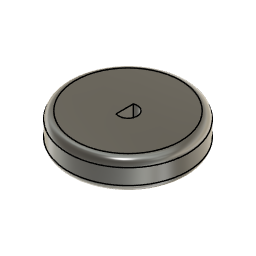
wheel v2 v1 (Autodesk Fusion 360 design; units mm, degrees)
Autodesk Fusion 360 part; units mm, degrees
note: some values were not read from the file. Set by a fixed rule: which sketch regions a step uses.
sketch "Sketch1" plane through (0, 0, 0) normal (0, 0, 1) x (1, 0, 0)
  circle A0 centre (0, 0) radius 10
  dimension "d1" = 20
  constraint coincident A0.centre origin
  measures "d1" diameter of A0
extrude "Extrude1" add sketch "Sketch1" along normal blind 5
fillet "Fillet1" radius 1.2 2 edges at (-9.3233, -3.6162, 5) (-9.3233, -3.6162, 0)
sketch "Sketch2" plane through (0, 0, 5) normal (0, 0, 1) x (-1, 0, 0)
  circle A0 centre (0, 0) radius 8.8
  circle A1 centre (0, 0) radius 1.55
  line L0 (0.55, 1.4491) -> (2.3002, 1.4491)
  line L1 (2.3002, 1.4491) -> (2.3002, -1.4465)
  line L2 (2.3002, -1.4465) -> (0.55, -1.4465)
  line L3 (0.55, -1.4465) -> (0.55, 1.4491)
  dimension "d6" = 3.1
  dimension "d7" = 0.55
  constraint concentric A0 A1
  constraint horizontal L0
  constraint vertical L1
  constraint horizontal L2
  constraint vertical L3
  constraint coincident A1 L0.start
  measures "d6" diameter of A1
  measures "d7" distance of A0.centre L3
extrude "Extrude2" cut sketch "Sketch2" against normal blind 50 contours A1 L3 picked at (-0.1277, 0.5002)
